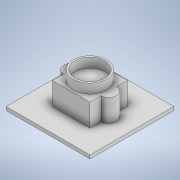
# Autodesk Inventor part: Camera Top
Saved by Autodesk Inventor 2020 (Build 240168000, 168)
## iProperties
Created: 2019-07-20
Part Number: Camera Top
Material: Generic
Document SubType Name: Modeling
Designer: Paul
Density: 1 g/cm^3
Appearance: Default
Author: Paul
Autodesk Inventor part; units mm, degrees
ref_plane "YZ Plane" through (0, 0, 0) normal (1, 0, 0) x (0, 1, 0)
ref_plane "XZ Plane" through (0, 0, 0) normal (0, 1, 0) x (-1, 0, 0)
ref_plane "XY Plane" through (0, 0, 0) normal (0, 0, 1) x (1, 0, 0)
sketch "Sketch1" plane through (0, 0, 0) normal (0, 1, 0) x (-1, 0, 0)
  line L0 (19, 19) -> (-19, 19)
  line L1 (-19, 19) -> (-19, -19)
  line L2 (-19, -19) -> (19, -19)
  line L3 (19, -19) -> (19, 19)
  line L4 (19, 19) -> (-19, -19) construction
  line L5 (-19, 19) -> (19, -19) construction
  point P0 (0, 0)
  dimension "d0" = 38
  dimension "d1" = 38
  constraints: 12 end point, 2 midpoint, 2 parallel, 1 horizontal, 1 perpendicular
  measures "d0" distance of L2.end L1.end
  measures "d1" distance of L1.end L0.end
extrude "Extrusion1" add sketch "Sketch1" along normal blind 1.6
sketch "Sketch2" plane through (0, 1.6, 0) normal (0, 1, 0) x (1, 0, 0)
  line L0 (-8.5, -8.5) -> (8.5, -8.5)
  line L1 (8.5, -8.5) -> (8.5, 8.5)
  line L2 (8.5, 8.5) -> (-8.5, 8.5)
  line L3 (-8.5, 8.5) -> (-8.5, -8.5)
  line L4 (-8.5, -8.5) -> (8.5, 8.5) construction
  line L5 (8.5, -8.5) -> (-8.5, 8.5) construction
  circle A0 centre (-8.5, 0) radius 3.5
  circle A1 centre (8.5, 0) radius 3.5
  point P0 (0, 0)
  point P1 (8.5, -3.5)
  point P2 (8.5, 3.5)
  point P3 (-8.5, 3.5)
  point P4 (-8.5, -3.5)
  dimension "d4" = 17
  dimension "d5" = 17
  dimension "d6" = 7
  dimension "d7" = 7
  constraints: 12 end point, 4 midpoint, 2 centre point, 2 parallel, 1 horizontal, 1 perpendicular
  measures "d4" distance of L2.end L1.end
  measures "d5" distance of L1.end L0.end
  measures "d6" diameter of A0
  measures "d7" diameter of A1
extrude "Extrusion2" add sketch "Sketch2" along normal blind 10.25
sketch "Sketch3" plane through (0, 11.85, 0) normal (0, 1, 0) x (1, 0, 0)
  circle A0 centre (0, 0) radius 7.6
  dimension "d10" = 15.2
  constraints: 1 centre point, 1 coincident
  measures "d10" diameter of A0
extrude "Extrusion3" add sketch "Sketch3" along normal blind 4.31
sketch "Sketch4" plane through (0, 16.16, 0) normal (0, 1, 0) x (1, 0, 0)
  circle A0 centre (0, 0) radius 6.83
  dimension "d13" = 13.66
  constraints: 1 centre point, 1 coincident
  measures "d13" diameter of A0
extrude "Extrusion4" cut sketch "Sketch4" against normal blind 4.31
sketch "Sketch5" plane through (0, 11.85, 0) normal (0, 1, 0) x (1, 0, 0)
  point P0 (0, 0)
body "Solid1"
